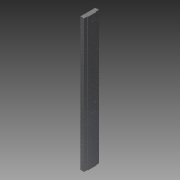
# Autodesk Inventor part: prowadnica 400mm pelny wysuw
Saved by Autodesk Inventor 2013 (Build 170138000, 138)
## iProperties
Created: 2014-05-06
Part Number: prowadnica 400mm pelny wysuw
Material: Generic
Document SubType Name: Modeling
Designer: Masta
Density: 1 g/cm^3
Author: Masta
Autodesk Inventor part; units mm, degrees
ref_plane "YZ Plane" through (0, 0, 0) normal (1, 0, 0) x (0, 1, 0)
ref_plane "XZ Plane" through (0, 0, 0) normal (0, 1, 0) x (-1, 0, 0)
ref_plane "XY Plane" through (0, 0, 0) normal (0, 0, 1) x (1, 0, 0)
sketch "Sketch1" plane through (0, 0, 0) normal (0, 0, 1) x (1, 0, 0)
  line L0 (0, 0) -> (11, 0)
  line L1 (11, 0) -> (11, 45)
  line L2 (11, 45) -> (0, 45)
  line L3 (0, 45) -> (0, 0)
  line L4 (0, 22.5) -> (11, 22.5) construction
  line L5 (11, 35) -> (12.7, 35)
  line L6 (12.7, 35) -> (12.7, 10)
  line L7 (12.7, 10) -> (11, 10)
  line L8 (11, 10) -> (11, 35)
  dimension "d0" = 11
  dimension "d1" = 45
  dimension "d2" = 1.7
  dimension "d3" = 25
  constraints: 18 end point, 4 parallel, 2 horizontal, 2 midpoint, 2 perpendicular, 1 point on line, 1 other
  measures "d0" distance of L2.end L1.end
  measures "d1" distance of L1.end L0.end
  measures "d2" distance of L5.start L5.end
  measures "d3" distance of L5.end L6.end
extrude "Extrusion1" add sketch "Sketch1" along normal blind 401
body "Solid1"
